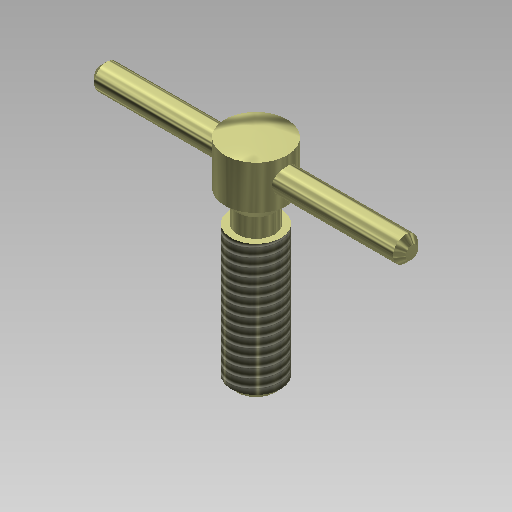
# Autodesk Inventor part: compression_ratio
Saved by Autodesk Inventor 2018.1 (Build 221171000, 171)
## iProperties
Created: 2013-08-26
Part Number: compression_ratio
Material: Generic
Document SubType Name: Modeling
Designer: Konstantin
Density: 1 g/cm^3
Appearance: Default
Mass: 0.295131 g
Surface Area: 3.81824 cm^2
Volume: 0.295131 cm^3
Author: Konstantin
Autodesk Inventor part; units mm, degrees
ref_plane "YZ Plane" through (0, 0, 0) normal (1, 0, 0) x (0, 1, 0)
ref_plane "XZ Plane" through (0, 0, 0) normal (0, 1, 0) x (-1, 0, 0)
ref_plane "XY Plane" through (0, 0, 0) normal (0, 0, 1) x (1, 0, 0)
sketch "Sketch1" plane through (0, 0, 0) normal (0, 0, 1) x (1, 0, 0)
  line L0 (2, 0) -> (2, 11)
  line L1 (2, 11) -> (1.5, 11)
  line L2 (0, 17.5) -> (0, 0)
  line L3 (2.5, 17) -> (2.5, 13.5)
  line L4 (1.5, 12.5) -> (2.5, 13.5)
  arc A0 (2.5, 17) -> (0, 17.5) centre (-0.8836, 6.5818) ccw
  line L5 (0, 0) -> (2, 0)
  line L6 (1.5, 11) -> (1.5, 12.5)
  constraints: 14 end point, 3 vertical, 2 horizontal, 2 perpendicular, 2 point on circle, 1 centre point, 1 parallel, 1 point on line, 2 other
revolve "Revolution1" add sketch "Sketch1" angle 360 about axis through (0, 17.5, 0) along (0, -1, 0)
chamfer "Chamfer1" distance 0.5 angle 45 1 edges at (-2, 0, 0)
thread "Thread1" size "M4x0.7" class "6g" standard "ISO Metric profile" full length
sketch "Sketch2" plane through (0, 0, 0) normal (1, 0, 0) x (0, 1, 0)
  circle A0 centre (15.25, 0) radius 1
  constraints: 1 centre point, 1 other
extrude "Extrusion1" add sketch "Sketch2" along normal mid plane 25
chamfer "Chamfer2" distance 0.5 angle 45 2 edges at (12.5, 14.25, 0) (-12.5, 14.25, 0)
body "Solid1"
